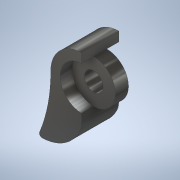
# Autodesk Inventor part: Part29
Saved by Autodesk Inventor 2021 (Build 250183000, 183)
## iProperties
Created: 2020-11-13
Part Number: Part29
Material: Liga de Nickel-Copper 400
Document SubType Name: Modeling
Designer: Lucas Moura
Density: 8.83 g/cm^3
Appearance: Cromado - Preto polido
Author: Lucas Moura
Autodesk Inventor part; units mm, degrees
ref_plane "YZ Plane" through (0, 0, 0) normal (1, 0, 0) x (0, 1, 0)
ref_plane "XZ Plane" through (0, 0, 0) normal (0, 1, 0) x (-1, 0, 0)
sketch "Sketch1" plane through (0, 0, 0) normal (0, 0, 1) x (1, 0, 0)
  line L0 (0, 0) -> (9.3091, 0)
  line L1 (9.3091, 0) -> (9.3091, 10)
  line L2 (9.3091, 10) -> (0, 10)
  line L3 (0, 10) -> (0, 0)
  circle A0 centre (4.6631, 6.6706) radius 2.3
  circle A1 centre (4.6631, 6.6706) radius 1
  line L4 (4.6312, 3.0206) -> (4.6312, 4.3708)
  line L5 (4.6312, 8.9703) -> (4.6312, 9.9704)
  arc A2 (4.6312, 9.9704) -> (1.3632, 6.6438) centre (4.6631, 6.6706) ccw
  arc A3 (4.639, 4.4786) -> (4.6548, 4.4787) centre (4.6389, 7.7786) ccw
  arc A4 (0, 0) -> (1.3632, 6.6438) centre (-14.8677, 6.5123) ccw
  arc A5 (0, 0) -> (4.6312, 3.0206) centre (0.3336, 4.5492) ccw
  dimension "d0" = 10
  dimension "d1" = 4.6
  dimension "d2" = 2
  constraints: 12 end point, 10 point on circle, 6 centre point, 2 coincident, 2 parallel, 1 collinear, 1 horizontal, 1 perpendicular, 1 tangent
  measures "d0" distance of L0.end L1.end
  measures "d1" diameter of A0
  measures "d2" diameter of A1
extrude "Extrusion1" add sketch "Sketch1" along normal blind 4 contours A4 A2 L5 A0 L4 A5 L0 | L0 A5 | A0
fillet "Fillet1" radius 2 1 edges at (4.6312, 3.0206, 2)
sketch "Sketch2" plane through (0, 0, 4) normal (0, 0, 1) x (1, 0, 0)
  line L0 (4.6312, 3.4171) -> (4.6312, 4.3708) projected
  arc A0 (4.6312, 4.3708) -> (4.6312, 8.9703) centre (4.6631, 6.6706) ccw projected
  line L1 (4.6312, 8.9703) -> (4.6312, 9.9704) projected
  arc A1 (4.6312, 9.9704) -> (1.3632, 6.6438) centre (4.6631, 6.6706) ccw projected
  circle A2 centre (4.6631, 6.6706) radius 1 projected
  circle A3 centre (4.6631, 6.6706) radius 2.3
  arc A4 (4.4253, 2.5332) -> (4.6312, 3.4171) centre (2.6312, 3.4171) ccw projected
  arc A5 (0, 0) -> (1.3632, 6.6438) centre (-14.8677, 6.5123) ccw projected
  arc A6 (0, 0) -> (4.4253, 2.5332) centre (0.3336, 4.5492) ccw projected
  constraints: 1 centre point, 1 coincident, 1 concentric
extrude "Extrusion2" cut sketch "Sketch2" against normal blind 1.3 contours A3 A0
sketch "Sketch3" plane through (0, 0, 0) normal (0, 0, -1) x (-1, 0, 0)
  arc A0 (-1.3632, 6.6438) -> (-4.6312, 9.9704) centre (-4.6631, 6.6706) ccw projected
  line L0 (-4.6312, 8.9703) -> (-4.6312, 9.9704) projected
  arc A1 (-4.6312, 8.9703) -> (-4.6312, 4.3708) centre (-4.6631, 6.6706) ccw projected
  line L1 (-4.6312, 3.4171) -> (-4.6312, 4.3708) projected
  circle A2 centre (-4.6631, 6.6706) radius 1 projected
  circle A3 centre (-4.6631, 6.6706) radius 2.3
  arc A4 (-4.6312, 3.4171) -> (-4.4253, 2.5332) centre (-2.6312, 3.4171) ccw projected
  arc A5 (-4.4253, 2.5332) -> (0, 0) centre (-0.3336, 4.5492) ccw projected
  arc A6 (-1.3632, 6.6438) -> (0, 0) centre (14.8677, 6.5123) ccw projected
  constraints: 1 centre point, 1 coincident, 1 concentric
extrude "Extrusion3" cut sketch "Sketch3" against normal blind 1.3 contours A3 A1
ref_plane "Work Plane5" through (4.6312, 3.8939, 0) normal (1, 0, 0) x (0, 0, -1)
sketch "Sketch6" plane through (4.6312, 3.8939, 0) normal (1, 0, 0) x (0, 0, -1)
  line L0 (0, -0.4768) -> (0, 0.4768) projected
  line L1 (0, 0.4768) -> (-1.3, 0.4768) projected
  line L2 (-1.3, 0.4768) -> (-2.7, 0.4768) projected
  line L3 (-2.7, 0.4768) -> (-4, 0.4768) projected
  line L4 (-4, -0.4768) -> (-4, 0.4768) projected
  circle A0 centre (-2, 0.1418) radius 0.275
  line L5 (-4, -0.4768) -> (-4, 0.4768) projected
  line L6 (0, -0.4768) -> (-4, -0.4768) projected
  line L7 (0, -0.4768) -> (0, 0.4768) projected
  line L8 (-4, 0.4768) -> (0, 0.4768)
  line L9 (0, 0.4768) -> (0, -0.1932)
  line L10 (0, -0.1932) -> (-4, -0.1932)
  line L11 (-4, -0.1932) -> (-4, 0.4768)
  line L12 (-4, 0.4768) -> (0, -0.1932) construction
  line L13 (-4, -0.1932) -> (0, 0.4768) construction
  point P0 (0, -3.8939)
  dimension "d22" = 0.55
  dimension "d26" = 0.67
  constraints: 12 end point, 2 parallel, 1 centre point, 1 horizontal, 1 midpoint, 1 perpendicular, 1 point on line
  measures "d22" diameter of A0
  measures "d26" distance of L8.end L9.end
extrude "Extrusion6" cut sketch "Sketch6" against normal blind 0.475 contours A0
fillet "Fillet2" radius 0.3 1 edges at (0, 0, 2)
body "Solid1"
